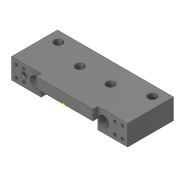
# Autodesk Inventor part: v2_front_ mount_2
Saved by Autodesk Inventor 2019 (Build 230136000, 136)
## iProperties
Created: 2017-06-19
Part Number: v2_front_ mount_2
Material: Aluminum 6061
Document SubType Name: Modeling
Designer: richp
Density: 2.7 g/cm^3
Appearance: Aluminum - Flat
Mass: 46.8621 g
Surface Area: 95.6149 cm^2
Volume: 17.3563 cm^3
front_mount_width: 2.840 in
Author: richp
Autodesk Inventor part; units mm, degrees
ref_plane "YZ Plane" through (0, 0, 0) normal (1, 0, 0) x (0, 1, 0)
ref_plane "XZ Plane" through (0, 0, 0) normal (0, 1, 0) x (-1, 0, 0)
sketch "Sketch1" plane through (0, 0, 0) normal (0, 0, 1) x (1, 0, 0)
  line L0 (-50.4952, 0) -> (50.4952, 0) projected
  line L1 (0, -8.89) -> (0, 8.89) projected
  line L2 (-36.068, 6.35) -> (36.068, 6.35)
  line L3 (36.068, 6.35) -> (36.068, -6.35)
  line L4 (36.068, -6.35) -> (-36.068, -6.35)
  line L5 (-36.068, -6.35) -> (-36.068, 6.35)
  point P0 (0, 0)
  point P1 (-21.209, 0)
  point P2 (21.209, 0)
  dimension "d0" = 42.418
  dimension "front_mount_width" = 72.136
  dimension "d2" = 12.7
  constraints: 8 end point, 2 parallel, 2 point on line, 1 horizontal, 1 perpendicular, 1 symmetric about line, 2 other
  measures "d0" distance of point (21.209, 0) point (-21.209, 0)
  measures "front_mount_width" distance between parallel lines of L3 L5
  measures "d2" distance between parallel lines of L4 L2
extrude "Extrusion1" add sketch "Sketch1" against normal blind 31.75
sketch "Sketch4" plane through (0, 0, 0) normal (0, 0, 1) x (1, 0, 0)
  line L0 (-50.4952, 0) -> (50.4952, 0) projected
  line L1 (0, -8.89) -> (0, 8.89) projected
  line L2 (-36.703, 6.35) -> (-17.653, 6.35)
  line L3 (-17.653, 6.35) -> (-17.653, -6.35)
  line L4 (-17.653, -6.35) -> (-36.703, -6.35)
  line L5 (-36.703, -6.35) -> (-36.703, 6.35)
  line L6 (36.703, 6.35) -> (17.653, 6.35)
  line L7 (17.653, 6.35) -> (17.653, -6.35)
  line L8 (17.653, -6.35) -> (36.703, -6.35)
  line L9 (36.703, -6.35) -> (36.703, 6.35)
  point P0 (0, 0)
  point P1 (-21.209, 0)
  dimension "d8" = 12.7
  dimension "d9" = 19.05
  dimension "d10" = 15.494
  constraints: 16 end point, 4 symmetric about line, 2 parallel, 1 horizontal, 1 perpendicular, 1 other
  measures "d8" distance between parallel lines of L4 L2
  measures "d9" distance between parallel lines of L3 L5
  measures "d10" distance from line of L5 point (-21.209, 0)
sketch "Sketch3" plane through (0, 0, 0) normal (0, 0, 1) x (1, 0, 0)
  line L0 (0, -8.89) -> (0, 8.89) projected
  line L1 (-50.4952, 0) -> (50.4952, 0) projected
  point P0 (0, 0)
  point P1 (-21.209, 0)
  point P2 (21.209, 0)
  point P3 (-14.097, 3.556)
  point P4 (-9.525, 3.556)
  point P5 (-14.097, -3.556)
  point P6 (-9.525, -3.556)
  point P7 (14.097, 3.556)
  point P8 (9.525, 3.556)
  point P9 (14.097, -3.556)
  point P10 (9.525, -3.556)
  dimension "d5" = 7.112
  dimension "d6" = 11.684
  dimension "d7" = 3.556
  constraints: 6 symmetric about line, 1 horizontal alignment
  measures "d5" horizontal distance of point (-14.097, 3.556) point (-21.209, 0)
  measures "d6" horizontal distance of point (-9.525, 3.556) point (-21.209, 0)
  measures "d7" distance from line of L1 point (-14.097, 3.556)
sketch "Sketch6" plane through (-36.068, 6.35, 0) normal (0, 1, 0) x (1, 0, 0)
  line L0 (93.218, 0) -> (-21.082, 0)
  line L1 (-21.082, 0) -> (-21.082, 31.75)
  line L2 (-21.082, 31.75) -> (93.218, 31.75)
  line L3 (93.218, 31.75) -> (93.218, 0)
  line L4 (0, 31.75) -> (72.136, 31.75) projected
  line L5 (0, 0) -> (72.136, 0) projected
  line L6 (36.068, 38.1) -> (36.068, -6.35) projected
  point P0 (36.068, 0)
  dimension "d27" = 57.15
  constraints: 8 end point, 2 collinear, 2 parallel, 1 horizontal, 1 perpendicular, 1 other
  measures "d27" distance between parallel lines of L3 L6
extrude "Extrusion3" [suppressed]
extrude "Extrusion2" cut sketch "Sketch4" against normal blind 3.175
hole "Hole1" [suppressed]
sketch "Sketch5" plane through (0, 0, 0) normal (0, 0, 1) x (1, 0, 0)
  point P0 (0, 0)
  point P1 (-21.209, 0)
  point P2 (21.209, 0)
hole "Hole2" at (-21.209, 0, 0) at (21.209, 0, 0) direction (0, 0, -1) diameter 6.35 depth 50.8 tip angle 118
sketch "Sketch8" plane through (57.15, 9.525, 0) normal (0, 1, 0) x (1, 0, 0)
  line L0 (-57.15, 30.48) -> (-57.15, -5.08) projected
  line L1 (-114.3, 0) -> (0, 0) projected
  point P0 (-57.15, 0)
  point P1 (-103.1875, 6.35)
  point P2 (-11.1125, 6.35)
  dimension "d39" = 46.0375
  dimension "d40" = 6.35
  constraints: 1 symmetric about line
  measures "d39" distance from line of point (-103.188, 6.35) L0
  measures "d40" distance from line of L1 point (-103.188, 6.35)
hole "Hole4" [suppressed]
sketch "Sketch9" plane through (57.15, 9.525, 0) normal (0, 1, 0) x (1, 0, 0)
  line L0 (-57.15, 30.48) -> (-57.15, -5.08) projected
  line L1 (-114.3, 0) -> (0, 0) projected
  point P0 (-57.15, 0)
  point P1 (-86.3092, 6.35)
  point P2 (-27.9908, 6.35)
  dimension "d48" = 58.3184
  dimension "d49" = 6.35
  constraints: 1 symmetric about line
  measures "d48" distance of point (-27.991, 6.35) point (-86.309, 6.35)
  measures "d49" distance from line of L1 point (-86.309, 6.35)
hole "Hole5" [suppressed]
sketch "Sketch10" plane through (-36.068, 6.35, 0) normal (0, 1, 0) x (1, 0, 0)
  line L0 (6.9088, 25.4) -> (6.9088, 8.89) construction
  line L1 (4.4196, 25.4) -> (4.4196, 8.89)
  line L2 (9.398, 8.89) -> (9.398, 25.4)
  arc A0 (9.398, 25.4) -> (4.4196, 25.4) centre (6.9088, 25.4) ccw
  arc A1 (4.4196, 8.89) -> (9.398, 8.89) centre (6.9088, 8.89) ccw
  line L3 (36.068, 38.1) -> (36.068, -6.35) projected
  line L4 (67.7164, 25.4) -> (67.7164, 8.89)
  line L5 (62.738, 8.89) -> (62.738, 25.4)
  arc A2 (67.7164, 25.4) -> (62.738, 25.4) centre (65.2272, 25.4) ccw
  arc A3 (62.738, 8.89) -> (67.7164, 8.89) centre (65.2272, 8.89) ccw
  line L6 (0, 0) -> (72.136, 0) projected
  line L7 (0, 31.75) -> (72.136, 31.75) projected
  point P0 (36.068, 0)
  point P1 (6.9088, 17.145)
  dimension "d57" = 58.3184
  dimension "d58" = 4.9784
  dimension "d59" = 8.89
  dimension "d60" = 6.35
  constraints: 12 end point, 8 point on circle, 6 symmetric about line, 4 centre point, 4 tangent, 1 midpoint, 1 parallel, 1 vertical, 2 other
  measures "d57" distance from line of A2.centre L0
  measures "d58" distance between parallel lines of L2 L1
  measures "d59" distance from line of L6 A3.centre
  measures "d60" distance from line of L7 A2.centre
extrude "Extrusion4" [suppressed]
sketch "Sketch12" plane through (0, 0, 0) normal (0, 0, 1) x (1, 0, 0)
  line L0 (-50.4952, 0) -> (50.4952, 0) projected
  line L1 (0, -8.89) -> (0, 8.89) projected
  point P0 (0, 0)
  point P1 (-21.209, 0)
  point P2 (-28.321, 3.556)
  point P3 (-32.893, 3.556)
  point P4 (-28.321, -3.556)
  point P5 (-32.893, -3.556)
  point P6 (28.321, 3.556)
  point P7 (32.893, 3.556)
  point P8 (32.893, -3.556)
  point P9 (28.321, -3.556)
  dimension "d63" = 7.112
  dimension "d64" = 11.684
  dimension "d65" = 3.556
  constraints: 6 symmetric about line, 1 horizontal alignment
  measures "d63" horizontal distance of point (-21.209, 0) point (-28.321, 3.556)
  measures "d64" horizontal distance of point (-21.209, 0) point (-32.893, 3.556)
  measures "d65" distance from line of L0 point (-28.321, 3.556)
hole "Hole6" at (-32.893, 3.556, 0) at (-28.321, 3.556, 0) at (-32.893, -3.556, 0) at (-28.321, -3.556, 0) at (28.321, 3.556, 0) at (32.893, 3.556, 0) at (28.321, -3.556, 0) at (32.893, -3.556, 0) direction (0, 0, -1) diameter 1.7018 depth 50.8 tip angle 118
sketch "Sketch13" plane through (-36.068, -6.35, -31.75) normal (0, -1, 0) x (1, 0, 0)
  line L0 (36.068, -6.35) -> (36.068, 38.1) projected
  line L1 (-14.4272, 31.75) -> (86.5632, 31.75) projected
  line L2 (53.721, 31.75) -> (18.415, 31.75) projected
  line L3 (21.7805, 31.75) -> (50.3555, 31.75)
  line L4 (50.3555, 31.75) -> (50.3555, 0)
  line L5 (50.3555, 0) -> (21.7805, 0)
  line L6 (21.7805, 0) -> (21.7805, 31.75)
  line L7 (72.136, 0) -> (0, 0) projected
  point P0 (36.068, 31.75)
  point P1 (36.068, 0)
  point P2 (20.712, 10.7844)
  dimension "d73" = 28.575
  constraints: 8 end point, 2 midpoint, 2 parallel, 1 horizontal, 1 perpendicular, 1 point on line, 1 other
  measures "d73" distance between parallel lines of L6 L4
extrude "Extrusion5" cut sketch "Sketch13" against normal blind 6.35
chamfer "Chamfer1" [suppressed]
sketch "Sketch14" plane through (-36.068, 6.35, -31.75) normal (0, 1, 0) x (1, 0, 0)
  line L0 (36.068, 6.35) -> (36.068, -38.1) projected
  line L1 (18.415, -31.75) -> (53.721, -31.75) projected
  point P0 (36.068, -31.75)
  point P1 (6.8724, -6.35)
  point P2 (65.2636, -6.35)
  dimension "d79" = 25.4
  constraints: 1 symmetric about line
  measures "d79" distance from line of L1 point (6.872, -6.35)
hole "Hole7" at (-29.1956, 6.35, -25.4) at (29.1956, 6.35, -25.4) direction (0, -1, 0) diameter 4.9784 depth 25.4 tip angle 118
sketch "Sketch15" plane through (-36.068, 6.35, -31.75) normal (0, 1, 0) x (1, 0, 0)
  line L0 (36.068, 6.35) -> (36.068, -38.1) construction
  line L1 (18.415, -31.75) -> (53.721, -31.75) projected
  point P0 (36.068, -31.75)
  point P1 (26.543, -12.7)
  point P2 (45.593, -12.7)
  dimension "d87" = 19.05
  dimension "d88" = 9.525
  constraints: 1 symmetric about line
  measures "d87" distance from line of L1 point (45.593, -12.7)
  measures "d88" distance from line of L0 point (45.593, -12.7)
hole "Hole8" at (-9.525, 6.35, -19.05) at (9.525, 6.35, -19.05) direction (0, -1, 0) diameter 4.9784 depth 14.9352 tip angle 118 clearance for "Flat Head Machine Screw (82)" size "#10" standard "Ansi Unified Screw Threads"
sketch "Sketch16" plane through (0, 0, 0) normal (0, 0, 1) x (1, 0, 0)
  line L0 (-14.2875, 0) -> (14.2875, 0) projected
  line L1 (0, -8.89) -> (0, 8.89) projected
  point P0 (0, 0)
  point P1 (0, 0)
  point P2 (0, 2.349)
  dimension "d96" = 2.349
  constraints: 1 point on line
  measures "d96" distance from line of L0 point (0, 2.349)
hole "Hole9" [suppressed]
sketch "Sketch17" plane through (0, 0, -3.175) normal (0, 0, 1) x (1, 0, 0)
  point P0 (0, 0)
  point P1 (-21.209, 0)
  point P2 (21.209, 0)
hole "Hole10" [suppressed]
sketch "Sketch18" plane through (-36.068, 6.35, -31.75) normal (0, 1, 0) x (1, 0, 0)
  line L0 (8.5979, -28.575) -> (6.8961, -28.575) projected
  line L1 (6.8961, 0) -> (8.5979, 0) projected
  line L2 (0, 0) -> (7.747, -28.575) construction
  line L3 (0, 0) -> (6.8961, 0) construction
  line L4 (7.747, -28.575) -> (1.27, 0)
  line L5 (7.0959, -28.575) -> (0.6189, 0) construction
  line L6 (-2.0115, -15.6677) -> (-0.7269, -12.645) construction
  line L7 (8.3345, -28.2943) -> (1.8575, 0.2807) construction
  point P0 (36.068, -31.75)
  dimension "d111" = 1.27
  dimension "d112" = 0.635
  constraints: 12 end point, 3 point on line, 2 symmetric about line, 1 horizontal, 1 midpoint, 1 parallel
  measures "d111" distance of L2.start L4.end
  measures "d112" distance between parallel lines of L4 L5
ref_plane "Work Plane1" through (-28.321, 6.35, -3.175) normal (-0.2211, 0, -0.9753) x (0, -1, 0)
sketch "Sketch19" plane through (-28.321, 6.35, -3.175) normal (-0.2211, 0, -0.9753) x (0, -1, 0)
  line L0 (6.35, 22.3275) -> (6.35, -76.1645) projected
  line L1 (0, 0) -> (6.35, 0) construction
  point P0 (6.35, -26.9185)
  constraints: 2 end point, 1 coincident, 1 perpendicular, 1 point on line
hole "Hole11" at (-28.321, 0, -3.175) direction (-0.2211, 0, -0.9753) diameter 2.032 end through all both
chamfer "Chamfer2" distance 0.762 angle 45 1 edges at (-28.321, 1.016, -3.175)
sketch "Sketch20" plane through (0, 0, 0) normal (0, 0, 1) x (1, 0, 0)
  line L0 (-14.2875, -6.35) -> (-36.068, -6.35) projected
  line L1 (-14.2875, -6.35) -> (-17.653, -6.35)
  line L2 (-17.653, -6.35) -> (-17.653, 6.35)
  line L3 (-17.653, 6.35) -> (-14.2875, 6.35)
  line L4 (-14.2875, 6.35) -> (-14.2875, -6.35)
  line L5 (14.2875, -6.35) -> (14.2875, 0) projected
  line L6 (17.653, 6.35) -> (36.068, 6.35) projected
  line L7 (14.2875, -6.35) -> (17.653, -6.35)
  line L8 (17.653, -6.35) -> (17.653, 6.35)
  line L9 (17.653, 6.35) -> (14.2875, 6.35)
  line L10 (14.2875, 6.35) -> (14.2875, -6.35)
  point P0 (0, 0)
  constraints: 16 end point, 4 parallel, 2 horizontal, 2 perpendicular
extrude "Extrusion6" [suppressed]
sketch "Sketch21" plane through (0, 0, 0) normal (0, 0, 1) x (1, 0, 0)
  line L0 (-17.653, 6.35) -> (-17.653, -6.35) projected
  line L1 (17.653, -6.35) -> (17.653, 6.35) projected
  line L2 (-17.653, -6.35) -> (17.653, -6.35)
  line L3 (17.653, -6.35) -> (17.653, 0)
  line L4 (17.653, 0) -> (-17.653, 0)
  line L5 (-17.653, 0) -> (-17.653, -6.35)
  point P0 (0, 0)
  constraints: 8 end point, 2 parallel, 1 horizontal, 1 midpoint, 1 perpendicular
extrude "Extrusion7" cut sketch "Sketch21" against normal blind 50.8
sketch "Sketch22" plane through (0, 0, 0) normal (0, 0, 1) x (1, 0, 0)
  point P0 (0, 0)
equation "\"d0\" = bearing_edge_distance"
equation "\"d5\" = hole1_setback"
equation "\"d6\" = hole2_setback"
equation "\"d7\" = hole_lateral"
equation "\"d63\" = hole1_setback"
equation "\"d64\" = hole2_setback"
equation "\"d65\" = hole_lateral"
equation "\"bearing_edge_distance\" = 42.418"
equation "\"hole1_setback\" = 7.112"
equation "\"hole2_setback\" = 11.684"
equation "\"hole_lateral\" = 3.556"
body "Solid1"
